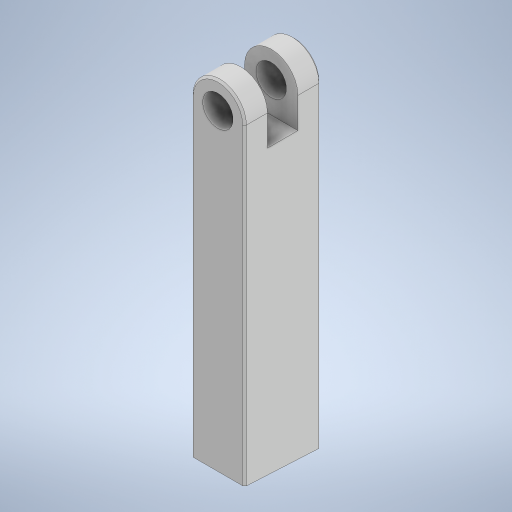
# Autodesk Inventor part: Schneidstempel
Saved by Autodesk Inventor 2024 (Build 280153000, 153)
## iProperties
Created: 2023-05-12
Part Number: Schneidstempel
Material: Generic
Document SubType Name: Modeling
Designer: Raj
Density: 1 g/cm^3
Appearance: Default
Author: Raj
Autodesk Inventor part; units mm, degrees
ref_plane "YZ Plane" through (0, 0, 0) normal (1, 0, 0) x (0, 1, 0)
ref_plane "XZ Plane" through (0, 0, 0) normal (0, 1, 0) x (-1, 0, 0)
ref_plane "XY Plane" through (0, 0, 0) normal (0, 0, 1) x (1, 0, 0)
sketch "Sketch1" plane through (0, 0, 0) normal (0, 1, 0) x (-1, 0, 0)
  arc A0 (7, 0) -> (-7, 0) centre (0, 0) ccw
  circle A1 centre (0, 0) radius 4
  line L0 (-7, 0) -> (-7, -83)
  line L1 (-7, -83) -> (7, -83)
  line L2 (7, -83) -> (7, 0)
  point P0 (0, -83)
  dimension "d0" = 14
  dimension "d1" = 8
  dimension "d2" = 83
  dimension "d3" = 14
  dimension "d4" = 83
  dimension "d5" = 0
  constraints: 6 end point, 2 centre point, 2 coincident, 2 point on circle, 1 midpoint, 1 perpendicular, 1 tangent
  measures "d0" diameter of A0
  measures "d1" diameter of A1
  measures "d2" distance of L0.start L0.end
  measures "d3" distance of L0.end L1.end
  measures "d4" distance from line of point (0, 0) L1
  measures "d5" horizontal distance of point (0, 0) point (0, -83)
extrude "Extrusion1" add sketch "Sketch1" along normal blind 20
sketch "Sketch2" plane through (7, 0, 0) normal (1, 0, 0) x (0, 0, -1)
  line L0 (0, 20) -> (83, 20) projected
  line L1 (83, 0) -> (83, 20) projected
  line L2 (83, 20) -> (81.9518, 0)
  line L3 (83, 20) -> (107.3414, 20) construction
  line L4 (83, 20) -> (83, 0)
  line L5 (83, 0) -> (81.9518, 0)
  line L6 (0, 0) -> (83, 0) projected
  dimension "d9" = 93
  constraints: 8 end point, 1 collinear, 1 horizontal, 1 point on line
  measures "d9" angle of L2 L3
extrude "Extrusion2" cut sketch "Sketch2" against normal through all
sketch "Sketch3" plane through (7, 0, 0) normal (1, 0, 0) x (0, 0, -1)
  line L0 (-7, 6) -> (8, 6)
  line L1 (8, 6) -> (8, 14)
  line L2 (8, 14) -> (-7, 14)
  line L3 (-7, 14) -> (-7, 6)
  line L4 (-7, 6) -> (8, 14) construction
  line L5 (8, 6) -> (-7, 14) construction
  point P0 (0, 0)
  point P1 (0.5, 10)
  dimension "d12" = 10
  dimension "d13" = 15
  dimension "d14" = 8
  dimension "d15" = 7
  constraints: 12 end point, 2 midpoint, 2 parallel, 1 horizontal, 1 perpendicular
  measures "d12" vertical distance of point (0.5, 10) point (0, 0)
  measures "d13" distance of L0.start L0.end
  measures "d14" distance of L2.end L0.start
  measures "d15" distance from line of point (0, 0) L3
extrude "Extrusion3" cut sketch "Sketch3" against normal through all
chamfer "Chamfer1" distance 0.5 angle 45 6 edges at (7, 0, -40.9759) (0, 0, 7) (-7, 0, -40.9759) (7, 20, -41.5) (0, 20, 7) (-7, 20, -41.5)
body "Solid1"
